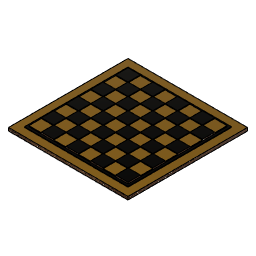
Chessboard (Autodesk Fusion 360 design; units mm, degrees)
Autodesk Fusion 360 part; units mm, degrees
sketch "Chessboard" plane through (0, 0, 0) normal (0, 1, 0) x (1, 0, 0)
  line L0 (-15.9564, 15.8169) -> (16.0436, 15.8169)
  line L1 (16.0436, 15.8169) -> (16.0436, -16.1831)
  line L2 (16.0436, -16.1831) -> (-15.9564, -16.1831)
  line L3 (-15.9564, -16.1831) -> (-15.9564, 15.8169)
  line L4 (16.7436, 16.5169) -> (16.7436, -16.8831)
  line L5 (16.7436, -16.8831) -> (-16.6564, -16.8831)
  line L6 (-16.6564, -16.8831) -> (-16.6564, 16.5169)
  line L7 (-16.6564, 16.5169) -> (16.7436, 16.5169)
  line L8 (19.3341, 19.1073) -> (19.3341, -19.4735)
  line L9 (19.3341, -19.4735) -> (-19.2468, -19.4735)
  line L10 (-19.2468, -19.4735) -> (-19.2468, 19.1073)
  line L11 (-19.2468, 19.1073) -> (19.3341, 19.1073)
  line L12 (-15.9564, 15.8169) -> (-11.9564, 15.8169)
  line L13 (-11.9564, 15.8169) -> (-7.9564, 15.8169)
  line L14 (-7.9564, 15.8169) -> (-3.9564, 15.8169)
  line L15 (-3.9564, 15.8169) -> (0.0436, 15.8169)
  line L16 (0.0436, 15.8169) -> (4.0436, 15.8169)
  line L17 (4.0436, 15.8169) -> (8.0436, 15.8169)
  line L18 (8.0436, 15.8169) -> (12.0436, 15.8169)
  line L19 (-15.9564, 15.8169) -> (-15.9564, 11.8169)
  line L20 (-15.9564, 11.8169) -> (-15.9564, 7.8169)
  line L21 (-15.9564, 7.8169) -> (-15.9564, 3.8169)
  line L22 (-15.9564, 3.8169) -> (-15.9564, -0.1831)
  line L23 (-15.9564, -0.1831) -> (-15.9564, -4.1831)
  line L24 (-15.9564, -4.1831) -> (-15.9564, -8.1831)
  line L25 (-15.9564, -8.1831) -> (-15.9564, -12.1831)
  line L26 (-11.9564, 15.8169) -> (-11.9564, -16.1831)
  line L27 (-7.9564, 15.8169) -> (-7.9564, -16.1831)
  line L28 (-3.9564, 15.8169) -> (-3.9564, -16.1831)
  line L29 (0.0436, 15.8169) -> (0.0436, -16.1831)
  line L30 (4.0436, 15.8169) -> (4.0436, -16.1831)
  line L31 (8.0436, 15.8169) -> (8.0436, -16.1831)
  line L32 (12.0436, 15.8169) -> (12.0436, -16.1831)
  line L33 (-15.9564, 11.8169) -> (16.0436, 11.8169)
  line L34 (-15.9564, 7.8169) -> (16.0436, 7.8169)
  line L35 (-15.9564, 3.8169) -> (16.0436, 3.8169)
  line L36 (-15.9564, -0.1831) -> (16.0436, -0.1831)
  line L37 (-15.9564, -4.1831) -> (16.0436, -4.1831)
  line L38 (-15.9564, -8.1831) -> (16.0436, -8.1831)
  line L39 (-15.9564, -12.1831) -> (16.0436, -12.1831)
  dimension "d3" = -0.7
  constraint horizontal L0
  constraint vertical L1
  constraint horizontal L2
  constraint vertical L3
  constraint perpendicular L3 L12
  constraint parallel L0 L13
  constraint coincident L0 L14.end
  constraint parallel L0 L15
  constraint parallel L0 L16
  constraint parallel L0 L17
  constraint parallel L0 L18
  constraint perpendicular L7 L19
  constraint parallel L3 L20
  constraint parallel L3 L21
  constraint parallel L3 L22
  constraint parallel L3 L23
  constraint parallel L3 L24
  constraint parallel L3 L25
  constraint coincident L2 L26.end
  constraint perpendicular L2 L26
  constraint perpendicular L13 L27
  constraint coincident L2 L28.end
  constraint perpendicular L2 L28
  constraint midpoint L2 L29.end
  constraint perpendicular L2 L29
  constraint coincident L2 L30.end
  constraint perpendicular L2 L30
  constraint coincident L2 L31.end
  constraint perpendicular L2 L31
  constraint coincident L2 L32.end
  constraint perpendicular L2 L32
  constraint coincident L1 L33.end
  constraint perpendicular L1 L33
  constraint perpendicular L32 L34
  constraint coincident L1 L35.end
  constraint perpendicular L1 L35
  constraint midpoint L1 L36.end
  constraint perpendicular L1 L36
  constraint coincident L1 L37.end
  constraint perpendicular L1 L37
  constraint perpendicular L32 L38
  constraint coincident L1 L39.end
  constraint perpendicular L1 L39
extrude "Extrude1" add sketch "Chessboard" along normal blind 1 contours L0 L3 L12 L19 L26 L33 | L0 L13 L26 L27 L33 | L3 L20 L26 L33 L34 | L0 L14 L27 L28 L33 | L26 L27 L33 L34 | L3 L21 L26 L34 L35 | L0 L15 L28 L29 L33 | L27 L28 L33 L34 | L26 L27 L34 L35 | L3 L22 L26 L35 L36 | L0 L16 L29 L30 L33 | L28 L29 L33 L34 | L27 L28 L34 L35 | L26 L27 L35 L36 | L3 L23 L26 L36 L37 | L0 L17 L30 L31 L33 | L29 L30 L33 L34 | L28 L29 L34 L35 | L27 L28 L35 L36 | L26 L27 L36 L37 | L3 L24 L26 L37 L38 | L0 L18 L31 L32 L33 | L30 L31 L33 L34 | L29 L30 L34 L35 | L28 L29 L35 L36 | L27 L28 L36 L37 | L26 L27 L37 L38 | L3 L25 L26 L38 L39 | L0 L1 L32 L33 | L31 L32 L33 L34 | L30 L31 L34 L35 | L29 L30 L35 L36 | L28 L29 L36 L37 | L27 L28 L37 L38 | L26 L27 L38 L39 | L2 L3 L26 L39 | L1 L32 L33 L34 | L31 L32 L34 L35 | L30 L31 L35 L36 | L29 L30 L36 L37 | L28 L29 L37 L38 | L27 L28 L38 L39 | L2 L26 L27 L39 | L1 L32 L34 L35 | L31 L32 L35 L36 | L30 L31 L36 L37 | L29 L30 L37 L38 | L28 L29 L38 L39 | L2 L27 L28 L39 | L1 L32 L35 L36 | L31 L32 L36 L37 | L30 L31 L37 L38 | L29 L30 L38 L39 | L2 L28 L29 L39 | L1 L32 L36 L37 | L31 L32 L37 L38 | L30 L31 L38 L39 | L2 L29 L30 L39 | L1 L32 L37 L38 | L31 L32 L38 L39 | L2 L30 L31 L39 | L1 L32 L38 L39 | L2 L31 L32 L39 | L1 L2 L32 L39 | L4 L5 L6 L7 | L8 L9 L10 L11
extrude "Extrude2" add sketch "Chessboard" along normal blind 1.2 contours L4 L5 L6 L7
extrude "Extrude3" add sketch "Chessboard" along normal blind 1.2 contours L0 L3 L12 L19 L26 L33 | L0 L14 L27 L28 L33 | L26 L27 L33 L34 | L3 L21 L26 L34 L35 | L0 L16 L29 L30 L33 | L28 L29 L33 L34 | L27 L28 L34 L35 | L26 L27 L35 L36 | L3 L23 L26 L36 L37 | L0 L18 L31 L32 L33 | L30 L31 L33 L34 | L29 L30 L34 L35 | L28 L29 L35 L36 | L27 L28 L36 L37 | L26 L27 L37 L38 | L3 L25 L26 L38 L39 | L1 L32 L33 L34 | L31 L32 L34 L35 | L30 L31 L35 L36 | L29 L30 L36 L37 | L28 L29 L37 L38 | L27 L28 L38 L39 | L2 L26 L27 L39 | L1 L32 L35 L36 | L31 L32 L36 L37 | L30 L31 L37 L38 | L29 L30 L38 L39 | L2 L28 L29 L39 | L1 L32 L37 L38 | L31 L32 L38 L39 | L2 L30 L31 L39 | L1 L2 L32 L39
extrude "Extrude4" add sketch "Chessboard" along normal blind 1.5 contours L0 L13 L26 L27 L33 | L3 L20 L26 L33 L34 | L0 L15 L28 L29 L33 | L27 L28 L33 L34 | L26 L27 L34 L35 | L3 L22 L26 L35 L36 | L0 L17 L30 L31 L33 | L29 L30 L33 L34 | L28 L29 L34 L35 | L27 L28 L35 L36 | L26 L27 L36 L37 | L3 L24 L26 L37 L38 | L0 L1 L32 L33 | L31 L32 L33 L34 | L30 L31 L34 L35 | L29 L30 L35 L36 | L28 L29 L36 L37 | L27 L28 L37 L38 | L26 L27 L38 L39 | L2 L3 L26 L39 | L1 L32 L34 L35 | L31 L32 L35 L36 | L30 L31 L36 L37 | L29 L30 L37 L38 | L28 L29 L38 L39 | L2 L27 L28 L39 | L1 L32 L36 L37 | L31 L32 L37 L38 | L30 L31 L38 L39 | L2 L29 L30 L39 | L1 L32 L38 L39 | L2 L31 L32 L39
extrude "Extrude5" add sketch "Chessboard" along normal blind 1 contours L0 L13 L26 L27 L33 | L3 L20 L26 L33 L34 | L0 L15 L28 L29 L33 | L27 L28 L33 L34 | L26 L27 L34 L35 | L3 L22 L26 L35 L36 | L0 L17 L30 L31 L33 | L29 L30 L33 L34 | L28 L29 L34 L35 | L27 L28 L35 L36 | L26 L27 L36 L37 | L3 L24 L26 L37 L38 | L0 L1 L32 L33 | L31 L32 L33 L34 | L30 L31 L34 L35 | L29 L30 L35 L36 | L28 L29 L36 L37 | L27 L28 L37 L38 | L26 L27 L38 L39 | L2 L3 L26 L39 | L1 L32 L34 L35 | L31 L32 L35 L36 | L30 L31 L36 L37 | L29 L30 L37 L38 | L28 L29 L38 L39 | L2 L27 L28 L39 | L1 L32 L36 L37 | L31 L32 L37 L38 | L30 L31 L38 L39 | L2 L29 L30 L39 | L1 L32 L38 L39 | L2 L31 L32 L39
extrude "Extrude6" add sketch "Chessboard" along normal blind 1.7 contours L0 L3 L12 L19 L26 L33 | L0 L14 L27 L28 L33 | L26 L27 L33 L34 | L3 L21 L26 L34 L35 | L0 L16 L29 L30 L33 | L28 L29 L33 L34 | L27 L28 L34 L35 | L26 L27 L35 L36 | L3 L23 L26 L36 L37 | L0 L18 L31 L32 L33 | L30 L31 L33 L34 | L29 L30 L34 L35 | L28 L29 L35 L36 | L27 L28 L36 L37 | L26 L27 L37 L38 | L3 L25 L26 L38 L39 | L1 L32 L33 L34 | L31 L32 L34 L35 | L30 L31 L35 L36 | L29 L30 L36 L37 | L28 L29 L37 L38 | L27 L28 L38 L39 | L2 L26 L27 L39 | L1 L32 L35 L36 | L31 L32 L36 L37 | L30 L31 L37 L38 | L29 L30 L38 L39 | L2 L28 L29 L39 | L1 L32 L37 L38 | L31 L32 L38 L39 | L2 L30 L31 L39 | L1 L2 L32 L39
named bodies: "Chessboard"
